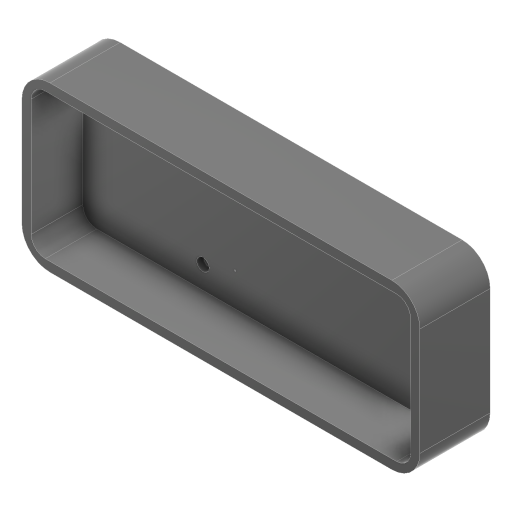
# Autodesk Inventor part: CASE_0
Saved by Autodesk Inventor 2023.2 (Build 272271000, 271)
## iProperties
Created: 2023-06-14
Part Number: CASE_0
Material: Generic
Document SubType Name: Modeling
Designer: samdi
Density: 1 g/cm^3
Appearance: Smooth - Black
Author: samdi
Autodesk Inventor part; units mm, degrees
ref_plane "YZ Plane" through (0, 0, 0) normal (1, 0, 0) x (0, 1, 0)
ref_plane "XZ Plane" through (0, 0, 0) normal (0, 1, 0) x (-1, 0, 0)
ref_plane "XY Plane" through (0, 0, 0) normal (0, 0, 1) x (1, 0, 0)
sketch "Sketch1" plane through (0, 0, 0) normal (0, 0, 1) x (1, 0, 0)
  line L0 (-16.1167, 9.6221) -> (-16.0287, 9.5557)
  line L1 (-16.2227, 9.6523) -> (-16.1167, 9.6221)
  line L2 (-16.3325, 9.6421) -> (-16.2227, 9.6523)
  line L3 (-16.4312, 9.593) -> (-16.3325, 9.6421)
  line L4 (-16.5055, 9.5115) -> (-16.4312, 9.593)
  line L5 (-16.0287, 9.5557) -> (-15.9707, 9.4619)
  line L6 (37.1652, -14.1251) -> (-36.8348, -14.1251)
  line L7 (37.1652, -14.1251) -> (-36.8348, -14.1251)
  line L8 (-13.126, 14.2536) -> (37.1652, 14.2536)
  line L9 (-13.126, 14.2536) -> (37.1652, 14.2536)
  circle A0 centre (21.1652, 10.2536) radius 1.35
  circle A1 centre (21.1652, 10.2536) radius 1.35
  line L10 (40.1652, 11.2536) -> (40.1652, -11.1251)
  line L11 (40.1652, 11.2536) -> (40.1652, -11.1251)
  line L12 (40.1463, 11.5895) -> (40.1652, 11.2536)
  line L13 (40.1463, 11.5895) -> (40.1652, 11.2536)
  line L14 (-16.4721, 8.3515) -> (-16.5301, 8.4452)
  line L15 (-16.4721, 8.3515) -> (-16.5301, 8.4452)
  line L16 (-15.971, 13.4619) -> (-15.9507, 13.3536)
  line L17 (-16.5507, 13.3536) -> (-16.5456, 13.4087)
  line L18 (-16.5507, 13.3536) -> (-16.5456, 13.4087)
  line L19 (-15.971, 13.4619) -> (-15.9507, 13.3536)
  line L20 (-16.5456, 13.4087) -> (-16.5058, 13.5115)
  line L21 (-16.5456, 13.4087) -> (-16.5058, 13.5115)
  line L22 (-16.029, 13.5557) -> (-15.971, 13.4619)
  line L23 (-16.029, 13.5557) -> (-15.971, 13.4619)
  line L24 (-16.117, 13.6221) -> (-16.029, 13.5557)
  line L25 (-16.117, 13.6221) -> (-16.029, 13.5557)
  line L26 (-16.223, 13.6523) -> (-16.117, 13.6221)
  line L27 (-16.223, 13.6523) -> (-16.117, 13.6221)
  line L28 (-16.3328, 13.6421) -> (-16.223, 13.6523)
  line L29 (-16.3328, 13.6421) -> (-16.223, 13.6523)
  line L30 (-16.5058, 13.5115) -> (-16.4315, 13.593)
  line L31 (-16.4315, 13.593) -> (-16.3328, 13.6421)
  line L32 (-16.4315, 13.593) -> (-16.3328, 13.6421)
  line L33 (-16.5058, 13.5115) -> (-16.4315, 13.593)
  line L34 (-39.1803, -12.9956) -> (-39.375, -12.7212)
  line L35 (-38.9562, -13.2464) -> (-39.1803, -12.9956)
  line L36 (-38.9562, -13.2464) -> (-39.1803, -12.9956)
  line L37 (-38.7053, -13.4706) -> (-38.9562, -13.2464)
  line L38 (-38.7053, -13.4706) -> (-38.9562, -13.2464)
  line L39 (-38.4309, -13.6653) -> (-38.7053, -13.4706)
  line L40 (-38.4309, -13.6653) -> (-38.7053, -13.4706)
  line L41 (-38.1365, -13.828) -> (-38.4309, -13.6653)
  line L42 (-38.1365, -13.828) -> (-38.4309, -13.6653)
  line L43 (-37.8257, -13.9568) -> (-38.1365, -13.828)
  line L44 (-37.8257, -13.9568) -> (-38.1365, -13.828)
  line L45 (-37.5024, -14.0499) -> (-37.8257, -13.9568)
  line L46 (-37.5024, -14.0499) -> (-37.8257, -13.9568)
  line L47 (-37.1707, -14.1062) -> (-37.5024, -14.0499)
  line L48 (-37.1707, -14.1062) -> (-37.5024, -14.0499)
  line L49 (-36.8348, -14.1251) -> (-37.1707, -14.1062)
  line L50 (-36.8348, -14.1251) -> (-37.1707, -14.1062)
  line L51 (-39.1803, -12.9956) -> (-39.375, -12.7212)
  line L52 (-27.681, 12.0452) -> (-27.7013, 12.1536)
  line L53 (-27.1013, 12.1536) -> (-27.1064, 12.0984)
  line L54 (-27.1013, 12.1536) -> (-27.1064, 12.0984)
  line L55 (-27.681, 12.0452) -> (-27.7013, 12.1536)
  line L56 (-27.1064, 12.0984) -> (-27.1462, 11.9956)
  line L57 (-27.1064, 12.0984) -> (-27.1462, 11.9956)
  line L58 (-27.623, 11.9515) -> (-27.681, 12.0452)
  line L59 (-27.623, 11.9515) -> (-27.681, 12.0452)
  line L60 (-27.535, 11.885) -> (-27.623, 11.9515)
  line L61 (-27.535, 11.885) -> (-27.623, 11.9515)
  line L62 (-27.429, 11.8548) -> (-27.535, 11.885)
  line L63 (-27.429, 11.8548) -> (-27.535, 11.885)
  line L64 (-27.1462, 11.9956) -> (-27.2205, 11.9142)
  line L65 (-27.3192, 11.865) -> (-27.429, 11.8548)
  line L66 (-27.3192, 11.865) -> (-27.429, 11.8548)
  line L67 (-27.2205, 11.9142) -> (-27.3192, 11.865)
  line L68 (-27.2205, 11.9142) -> (-27.3192, 11.865)
  line L69 (-27.1462, 11.9956) -> (-27.2205, 11.9142)
  line L70 (-27.7013, 12.1536) -> (-27.7013, 13.3536)
  line L71 (-27.1013, 13.3536) -> (-27.1013, 12.1536)
  line L72 (-27.7013, 12.1536) -> (-27.7013, 13.3536)
  line L73 (-27.1013, 13.3536) -> (-27.1013, 12.1536)
  line L74 (-27.7013, 13.3536) -> (-27.6962, 13.4087)
  line L75 (-27.7013, 13.3536) -> (-27.6962, 13.4087)
  line L76 (-27.1216, 13.4619) -> (-27.1013, 13.3536)
  line L77 (-27.1216, 13.4619) -> (-27.1013, 13.3536)
  line L78 (-27.6962, 13.4087) -> (-27.6564, 13.5115)
  line L79 (-27.6962, 13.4087) -> (-27.6564, 13.5115)
  line L80 (-27.1796, 13.5557) -> (-27.1216, 13.4619)
  line L81 (-27.1796, 13.5557) -> (-27.1216, 13.4619)
  line L82 (-27.2676, 13.6221) -> (-27.1796, 13.5557)
  line L83 (-27.2676, 13.6221) -> (-27.1796, 13.5557)
  line L84 (-27.6564, 13.5115) -> (-27.5821, 13.593)
  line L85 (-27.6564, 13.5115) -> (-27.5821, 13.593)
  line L86 (-27.5821, 13.593) -> (-27.4834, 13.6421)
  line L87 (-27.5821, 13.593) -> (-27.4834, 13.6421)
  line L88 (-27.4834, 9.6421) -> (-27.3736, 9.6523)
  line L89 (-27.4834, 9.6421) -> (-27.3736, 9.6523)
  line L90 (-27.3736, 9.6523) -> (-27.2676, 9.6221)
  line L91 (-27.6564, 9.5115) -> (-27.5821, 9.593)
  line L92 (-27.6962, 9.4087) -> (-27.6564, 9.5115)
  line L93 (-27.3736, 9.6523) -> (-27.2676, 9.6221)
  line L94 (-16.5507, 12.1536) -> (-16.5507, 13.3536)
  line L95 (-16.5304, 12.0452) -> (-16.5507, 12.1536)
  line L96 (-16.4724, 11.9515) -> (-16.5304, 12.0452)
  line L97 (-15.9507, 13.3536) -> (-15.9507, 12.1536)
  line L98 (-15.9507, 12.1536) -> (-15.9558, 12.0984)
  line L99 (-16.5507, 12.1536) -> (-16.5507, 13.3536)
  line L100 (-15.9507, 13.3536) -> (-15.9507, 12.1536)
  line L101 (-15.9507, 12.1536) -> (-15.9558, 12.0984)
  line L102 (-16.5304, 12.0452) -> (-16.5507, 12.1536)
  line L103 (-15.9558, 12.0984) -> (-15.9956, 11.9956)
  line L104 (-16.3844, 11.885) -> (-16.4724, 11.9515)
  line L105 (-16.3844, 11.885) -> (-16.4724, 11.9515)
  line L106 (-16.2784, 11.8548) -> (-16.3844, 11.885)
  line L107 (-16.2784, 11.8548) -> (-16.3844, 11.885)
  line L108 (-16.1686, 11.865) -> (-16.2784, 11.8548)
  line L109 (-16.1686, 11.865) -> (-16.2784, 11.8548)
  line L110 (-15.9956, 11.9956) -> (-16.0699, 11.9142)
  line L111 (-15.9956, 11.9956) -> (-16.0699, 11.9142)
  line L112 (-16.0699, 11.9142) -> (-16.1686, 11.865)
  line L113 (-16.0699, 11.9142) -> (-16.1686, 11.865)
  line L114 (-15.9558, 12.0984) -> (-15.9956, 11.9956)
  line L115 (-15.9504, 8.5536) -> (-15.9555, 8.4984)
  line L116 (-15.9504, 9.3536) -> (-15.9504, 8.5536)
  line L117 (-15.9707, 9.4619) -> (-15.9504, 9.3536)
  line L118 (-16.0287, 9.5557) -> (-15.9707, 9.4619)
  line L119 (-16.1167, 9.6221) -> (-16.0287, 9.5557)
  line L120 (-16.2227, 9.6523) -> (-16.1167, 9.6221)
  line L121 (-16.5453, 9.4087) -> (-16.5055, 9.5115)
  line L122 (-16.5504, 9.3536) -> (-16.5453, 9.4087)
  line L123 (-16.5504, 8.5536) -> (-16.5504, 9.3536)
  line L124 (-16.3325, 9.6421) -> (-16.2227, 9.6523)
  line L125 (-16.4312, 9.593) -> (-16.3325, 9.6421)
  line L126 (-15.9707, 9.4619) -> (-15.9504, 9.3536)
  line L127 (-15.9504, 9.3536) -> (-15.9504, 8.5536)
  line L128 (-15.9504, 8.5536) -> (-15.9555, 8.4984)
  line L129 (-16.5055, 9.5115) -> (-16.4312, 9.593)
  line L130 (-16.5453, 9.4087) -> (-16.5055, 9.5115)
  line L131 (-16.5504, 9.3536) -> (-16.5453, 9.4087)
  line L132 (-16.5504, 8.5536) -> (-16.5504, 9.3536)
  line L133 (-17.226, 8.4536) -> (-17.226, 14.2536)
  line L134 (-26.426, 14.2536) -> (-26.426, 8.4536)
  line L135 (-26.426, 14.2536) -> (-26.426, 8.4536)
  line L136 (-17.226, 8.4536) -> (-17.226, 14.2536)
  line L137 (-17.226, 14.2536) -> (-13.126, 14.2536)
  line L138 (-17.226, 14.2536) -> (-13.126, 14.2536)
  line L139 (-16.4724, 11.9515) -> (-16.5304, 12.0452)
  line L140 (-26.426, 8.4536) -> (-17.226, 8.4536)
  line L141 (-26.426, 8.4536) -> (-17.226, 8.4536)
  circle A2 centre (-14.8348, -10.7464) radius 1.35
  circle A3 centre (-14.8348, -10.7464) radius 1.35
  circle A4 centre (-35.8348, 10.2536) radius 1.35
  line L142 (-37.5024, 14.1784) -> (-37.1707, 14.2347)
  line L143 (-37.8257, 14.0852) -> (-37.5024, 14.1784)
  line L144 (-36.8348, 14.2536) -> (-29.926, 14.2536)
  line L145 (-36.8348, 14.2536) -> (-29.926, 14.2536)
  circle A5 centre (-35.8348, 10.2536) radius 1.35
  line L146 (-37.1707, 14.2347) -> (-36.8348, 14.2536)
  line L147 (-37.1707, 14.2347) -> (-36.8348, 14.2536)
  line L148 (-37.5024, 14.1784) -> (-37.1707, 14.2347)
  line L149 (-37.8257, 14.0852) -> (-37.5024, 14.1784)
  line L150 (-27.681, 8.4452) -> (-27.7013, 8.5536)
  line L151 (-27.7013, 8.5536) -> (-27.7013, 9.3536)
  line L152 (-27.1216, 9.4619) -> (-27.1013, 9.3536)
  line L153 (-27.1013, 9.3536) -> (-27.1013, 8.5536)
  line L154 (-27.1796, 9.5557) -> (-27.1216, 9.4619)
  line L155 (-27.1013, 8.5536) -> (-27.1064, 8.4984)
  line L156 (-27.1064, 8.4984) -> (-27.1462, 8.3956)
  line L157 (-27.2676, 9.6221) -> (-27.1796, 9.5557)
  line L158 (-27.7013, 9.3536) -> (-27.6962, 9.4087)
  line L159 (-27.5821, 9.593) -> (-27.4834, 9.6421)
  line L160 (-27.2676, 9.6221) -> (-27.1796, 9.5557)
  line L161 (-27.6564, 9.5115) -> (-27.5821, 9.593)
  line L162 (-27.1796, 9.5557) -> (-27.1216, 9.4619)
  line L163 (-27.6962, 9.4087) -> (-27.6564, 9.5115)
  line L164 (-27.1216, 9.4619) -> (-27.1013, 9.3536)
  line L165 (-27.7013, 9.3536) -> (-27.6962, 9.4087)
  line L166 (-27.1013, 9.3536) -> (-27.1013, 8.5536)
  line L167 (-27.7013, 8.5536) -> (-27.7013, 9.3536)
  line L168 (-27.681, 8.4452) -> (-27.7013, 8.5536)
  line L169 (-27.623, 8.3515) -> (-27.681, 8.4452)
  line L170 (-27.623, 8.3515) -> (-27.681, 8.4452)
  line L171 (-27.5821, 9.593) -> (-27.4834, 9.6421)
  line L172 (-27.1064, 8.4984) -> (-27.1462, 8.3956)
  line L173 (-27.1462, 8.3956) -> (-27.2205, 8.3142)
  line L174 (-27.1462, 8.3956) -> (-27.2205, 8.3142)
  line L175 (-27.535, 8.285) -> (-27.623, 8.3515)
  line L176 (-27.535, 8.285) -> (-27.623, 8.3515)
  line L177 (-27.2205, 8.3142) -> (-27.3192, 8.265)
  line L178 (-27.2205, 8.3142) -> (-27.3192, 8.265)
  line L179 (-27.429, 8.2548) -> (-27.535, 8.285)
  line L180 (-27.429, 8.2548) -> (-27.535, 8.285)
  line L181 (-27.3192, 8.265) -> (-27.429, 8.2548)
  line L182 (-27.3192, 8.265) -> (-27.429, 8.2548)
  line L183 (-27.1013, 8.5536) -> (-27.1064, 8.4984)
  line L184 (-27.3736, 13.6523) -> (-27.2676, 13.6221)
  line L185 (-27.4834, 13.6421) -> (-27.3736, 13.6523)
  line L186 (-27.4834, 13.6421) -> (-27.3736, 13.6523)
  line L187 (-29.926, 14.2536) -> (-26.426, 14.2536)
  line L188 (-29.926, 14.2536) -> (-26.426, 14.2536)
  line L189 (-27.3736, 13.6523) -> (-27.2676, 13.6221)
  circle A6 centre (-7.9777, -8.4364) radius 0.15
  circle A7 centre (-7.9777, -8.4364) radius 0.15
  line L190 (-15.9555, 8.4984) -> (-15.9953, 8.3956)
  line L191 (-15.9555, 8.4984) -> (-15.9953, 8.3956)
  line L192 (-15.9953, 8.3956) -> (-16.0696, 8.3142)
  line L193 (-15.9953, 8.3956) -> (-16.0696, 8.3142)
  line L194 (-16.0696, 8.3142) -> (-16.1683, 8.265)
  line L195 (-16.0696, 8.3142) -> (-16.1683, 8.265)
  line L196 (-16.1683, 8.265) -> (-16.2781, 8.2548)
  line L197 (-16.1683, 8.265) -> (-16.2781, 8.2548)
  line L198 (-16.2781, 8.2548) -> (-16.3841, 8.285)
  line L199 (-16.2781, 8.2548) -> (-16.3841, 8.285)
  line L200 (-16.3841, 8.285) -> (-16.4721, 8.3515)
  line L201 (-16.3841, 8.285) -> (-16.4721, 8.3515)
  line L202 (-16.5301, 8.4452) -> (-16.5504, 8.5536)
  line L203 (-16.5301, 8.4452) -> (-16.5504, 8.5536)
  line L204 (-39.8348, -11.1251) -> (-39.8348, 11.2536)
  line L205 (-39.8348, -11.1251) -> (-39.8348, 11.2536)
  line L206 (39.0356, 13.5991) -> (39.2865, 13.3749)
  line L207 (39.0356, 13.5991) -> (39.2865, 13.3749)
  line L208 (38.7613, 13.7937) -> (39.0356, 13.5991)
  line L209 (38.7613, 13.7937) -> (39.0356, 13.5991)
  line L210 (38.4668, 13.9565) -> (38.7613, 13.7937)
  line L211 (38.4668, 13.9565) -> (38.7613, 13.7937)
  line L212 (38.156, 14.0852) -> (38.4668, 13.9565)
  line L213 (38.156, 14.0852) -> (38.4668, 13.9565)
  line L214 (37.8327, 14.1784) -> (38.156, 14.0852)
  line L215 (37.8327, 14.1784) -> (38.156, 14.0852)
  line L216 (37.5011, 14.2347) -> (37.8327, 14.1784)
  line L217 (37.5011, 14.2347) -> (37.8327, 14.1784)
  line L218 (37.1652, 14.2536) -> (37.5011, 14.2347)
  line L219 (37.1652, 14.2536) -> (37.5011, 14.2347)
  line L220 (39.2865, 13.3749) -> (39.5107, 13.124)
  line L221 (39.2865, 13.3749) -> (39.5107, 13.124)
  line L222 (39.5107, 13.124) -> (39.7053, 12.8497)
  line L223 (39.5107, 13.124) -> (39.7053, 12.8497)
  line L224 (39.7053, 12.8497) -> (39.8681, 12.5552)
  line L225 (39.8681, 12.5552) -> (39.9968, 12.2444)
  line L226 (39.8681, 12.5552) -> (39.9968, 12.2444)
  line L227 (39.9968, 12.2444) -> (40.0899, 11.9211)
  line L228 (39.9968, 12.2444) -> (40.0899, 11.9211)
  line L229 (40.0899, 11.9211) -> (40.1463, 11.5895)
  line L230 (40.0899, 11.9211) -> (40.1463, 11.5895)
  line L231 (39.7053, 12.8497) -> (39.8681, 12.5552)
  line L232 (-39.8348, 11.2536) -> (-39.816, 11.5895)
  line L233 (-39.816, 11.5895) -> (-39.7596, 11.9211)
  line L234 (-38.1365, 13.9565) -> (-37.8257, 14.0852)
  line L235 (-38.4309, 13.7937) -> (-38.1365, 13.9565)
  line L236 (-38.7053, 13.5991) -> (-38.4309, 13.7937)
  line L237 (-38.9562, 13.3749) -> (-38.7053, 13.5991)
  line L238 (-39.1803, 13.124) -> (-38.9562, 13.3749)
  line L239 (-39.375, 12.8497) -> (-39.1803, 13.124)
  line L240 (-39.5377, 12.5552) -> (-39.375, 12.8497)
  line L241 (-39.6665, 12.2444) -> (-39.5377, 12.5552)
  line L242 (-39.7596, 11.9211) -> (-39.6665, 12.2444)
  line L243 (-38.1365, 13.9565) -> (-37.8257, 14.0852)
  line L244 (-38.4309, 13.7937) -> (-38.1365, 13.9565)
  line L245 (-38.7053, 13.5991) -> (-38.4309, 13.7937)
  line L246 (-38.9562, 13.3749) -> (-38.7053, 13.5991)
  line L247 (-39.1803, 13.124) -> (-38.9562, 13.3749)
  line L248 (-39.375, 12.8497) -> (-39.1803, 13.124)
  line L249 (-39.5377, 12.5552) -> (-39.375, 12.8497)
  line L250 (-39.6665, 12.2444) -> (-39.5377, 12.5552)
  line L251 (-39.7596, 11.9211) -> (-39.6665, 12.2444)
  line L252 (-39.8348, 11.2536) -> (-39.816, 11.5895)
  line L253 (-39.816, 11.5895) -> (-39.7596, 11.9211)
  line L254 (-39.5377, -12.4268) -> (-39.6665, -12.1159)
  line L255 (-39.375, -12.7212) -> (-39.5377, -12.4268)
  line L256 (-39.375, -12.7212) -> (-39.5377, -12.4268)
  line L257 (-39.5377, -12.4268) -> (-39.6665, -12.1159)
  line L258 (-39.6665, -12.1159) -> (-39.7596, -11.7927)
  line L259 (-39.7596, -11.7927) -> (-39.816, -11.461)
  line L260 (-39.7596, -11.7927) -> (-39.816, -11.461)
  line L261 (-39.816, -11.461) -> (-39.8348, -11.1251)
  line L262 (-39.816, -11.461) -> (-39.8348, -11.1251)
  line L263 (-39.6665, -12.1159) -> (-39.7596, -11.7927)
  line L264 (37.5011, -14.1062) -> (37.1652, -14.1251)
  line L265 (38.7613, -13.6653) -> (38.4668, -13.828)
  line L266 (38.7613, -13.6653) -> (38.4668, -13.828)
  line L267 (39.5107, -12.9956) -> (39.2865, -13.2464)
  line L268 (39.9968, -12.1159) -> (39.8681, -12.4268)
  line L269 (40.1652, -11.1251) -> (40.1463, -11.461)
  line L270 (40.1652, -11.1251) -> (40.1463, -11.461)
  line L271 (40.1463, -11.461) -> (40.0899, -11.7927)
  line L272 (40.1463, -11.461) -> (40.0899, -11.7927)
  line L273 (40.0899, -11.7927) -> (39.9968, -12.1159)
  line L274 (40.0899, -11.7927) -> (39.9968, -12.1159)
  line L275 (39.9968, -12.1159) -> (39.8681, -12.4268)
  line L276 (39.8681, -12.4268) -> (39.7053, -12.7212)
  line L277 (39.8681, -12.4268) -> (39.7053, -12.7212)
  line L278 (39.7053, -12.7212) -> (39.5107, -12.9956)
  line L279 (39.7053, -12.7212) -> (39.5107, -12.9956)
  line L280 (39.5107, -12.9956) -> (39.2865, -13.2464)
  line L281 (39.2865, -13.2464) -> (39.0356, -13.4706)
  line L282 (39.2865, -13.2464) -> (39.0356, -13.4706)
  line L283 (39.0356, -13.4706) -> (38.7613, -13.6653)
  line L284 (39.0356, -13.4706) -> (38.7613, -13.6653)
  line L285 (38.4668, -13.828) -> (38.156, -13.9568)
  line L286 (38.4668, -13.828) -> (38.156, -13.9568)
  line L287 (38.156, -13.9568) -> (37.8327, -14.0499)
  line L288 (37.8327, -14.0499) -> (37.5011, -14.1062)
  line L289 (37.8327, -14.0499) -> (37.5011, -14.1062)
  line L290 (37.5011, -14.1062) -> (37.1652, -14.1251)
  line L291 (38.156, -13.9568) -> (37.8327, -14.0499)
  line L292 (-36.5, 17.5) -> (36.5, 17.5)
  line L293 (42.5, 11.5) -> (42.5, -11.5)
  line L294 (36.5, -17.5) -> (-36.5, -17.5)
  line L295 (-42.5, -11.5) -> (-42.5, 11.5)
  line L296 (-42.5, 17.5) -> (42.5, -17.5) construction
  line L297 (42.5, 17.5) -> (-42.5, -17.5) construction
  arc A8 (-36.5, 17.5) -> (-42.5, 11.5) centre (-36.5, 11.5) ccw
  arc A9 (-42.5, -11.5) -> (-36.5, -17.5) centre (-36.5, -11.5) ccw
  arc A10 (36.5, -17.5) -> (42.5, -11.5) centre (36.5, -11.5) ccw
  arc A11 (42.5, 11.5) -> (36.5, 17.5) centre (36.5, 11.5) ccw
  line L298 (37.5, 15.5) -> (-37.5, 15.5)
  line L299 (-40.5, 12.5) -> (-40.5, -12.5)
  line L300 (-37.5, -15.5) -> (37.5, -15.5)
  line L301 (40.5, -12.5) -> (40.5, 12.5)
  line L302 (40.5, 15.5) -> (-40.5, -15.5) construction
  line L303 (-40.5, 15.5) -> (40.5, -15.5) construction
  arc A12 (-40.5, -12.5) -> (-37.5, -15.5) centre (-37.5, -12.5) ccw
  arc A13 (-37.5, 15.5) -> (-40.5, 12.5) centre (-37.5, 12.5) ccw
  arc A14 (40.5, 12.5) -> (37.5, 15.5) centre (37.5, 12.5) ccw
  arc A15 (37.5, -15.5) -> (40.5, -12.5) centre (37.5, -12.5) ccw
  point P0 (0, 0)
  dimension "d2" = 85
  dimension "d3" = 35
  dimension "d4" = 6
  dimension "d5" = 81
  dimension "d6" = 31
  dimension "d7" = 3
  dimension "d8" = 3
  constraints: 608 end point, 16 centre point, 16 point on circle, 16 point on line, 16 tangent, 5 equal radius, 4 midpoint, 4 parallel, 2 horizontal, 2 perpendicular
  measures "d2" distance of L296.end L297.end
  measures "d3" distance of L297.start L296.end
  measures "d4" radius of A8
  measures "d5" distance of L303.end L302.end
  measures "d6" distance of L302.end L303.start
  measures "d7" radius of A12
  measures "d8" radius of A13
extrude "Extrusion1" add sketch "Sketch1" along normal blind 2.5 contours L0 L5 L117 L116 L115 L190 L192 L194 L196 L198 L200 L14 L202 L123 L122 L121 L4 L3 L2 L1 | L6 L49 L47 L45 L43 L41 L39 L37 L35 L34 L255 L254 L258 L259 L261 L204 L232 L233 L242 L241 L240 L239 L238 L237 L236 L235 L234 L143 L142 L146 L144 L187 L134 L140 L133 L137 L8 L218 L216 L214 L212 L210 L208 L206 L220 L222 L224 L225 L227 L229 L12 L10 L269 L271 L273 L268 L276 L278 L267 L281 L283 L265 L285 L287 L288 L264 | A0 | L16 L97 L98 L103 L110 L112 L108 L106 L104 L96 L95 L94 L17 L20 L30 L31 L28 L26 L24 L22 | L52 L70 L74 L78 L84 L86 L185 L184 L82 L80 L76 L71 L53 L56 L64 L67 L65 L62 L60 L58 | L88 L90 L157 L154 L152 L153 L155 L156 L173 L177 L181 L179 L175 L169 L150 L151 L158 L92 L91 L159 | A2 | A4 | A6 | L292 A11 L293 A10 L294 A9 L295 A8 | A14 L301 A15 L300 A12 L299 A13 L298
extrude "Extrusion2" add sketch "Sketch1" along normal blind 15 contours L292 A11 L293 A10 L294 A9 L295 A8
extrude "Extrusion3" add sketch "Sketch1" along normal blind 4 contours L0 L5 L117 L116 L115 L190 L192 L194 L196 L198 L200 L14 L202 L123 L122 L121 L4 L3 L2 L1 | L6 L49 L47 L45 L43 L41 L39 L37 L35 L34 L255 L254 L258 L259 L261 L204 L232 L233 L242 L241 L240 L239 L238 L237 L236 L235 L234 L143 L142 L146 L144 L187 L134 L140 L133 L137 L8 L218 L216 L214 L212 L210 L208 L206 L220 L222 L224 L225 L227 L229 L12 L10 L269 L271 L273 L268 L276 L278 L267 L281 L283 L265 L285 L287 L288 L264 | L16 L97 L98 L103 L110 L112 L108 L106 L104 L96 L95 L94 L17 L20 L30 L31 L28 L26 L24 L22 | L52 L70 L74 L78 L84 L86 L185 L184 L82 L80 L76 L71 L53 L56 L64 L67 L65 L62 L60 L58 | L88 L90 L157 L154 L152 L153 L155 L156 L173 L177 L181 L179 L175 L169 L150 L151 L158 L92 L91 L159 | A14 L301 A15 L300 A12 L299 A13 L298
sketch "Sketch3" plane through (0, 0, 15) normal (0, 0, 1) x (1, 0, 0)
  line L0 (-36.5, -17.5) -> (36.5, -17.5) projected
  arc A0 (36.5, -17.5) -> (42.5, -11.5) centre (36.5, -11.5) ccw projected
  line L1 (42.5, -11.5) -> (42.5, 11.5) projected
  arc A1 (42.5, 11.5) -> (36.5, 17.5) centre (36.5, 11.5) ccw projected
  line L2 (36.5, 17.5) -> (-36.5, 17.5) projected
  arc A2 (-36.5, 17.5) -> (-42.5, 11.5) centre (-36.5, 11.5) ccw projected
  line L3 (-42.5, 11.5) -> (-42.5, -11.5) projected
  arc A3 (-42.5, -11.5) -> (-36.5, -17.5) centre (-36.5, -11.5) ccw projected
  arc A4 (40.5, 12.5) -> (37.5, 15.5) centre (37.5, 12.5) ccw projected
  line L4 (40.5, 12.5) -> (40.5, -12.5) projected
  arc A5 (37.5, -15.5) -> (40.5, -12.5) centre (37.5, -12.5) ccw projected
  line L5 (37.5, -15.5) -> (-37.5, -15.5) projected
  arc A6 (-40.5, -12.5) -> (-37.5, -15.5) centre (-37.5, -12.5) ccw projected
  line L6 (-40.5, -12.5) -> (-40.5, 12.5) projected
  arc A7 (-37.5, 15.5) -> (-40.5, 12.5) centre (-37.5, 12.5) ccw projected
  line L7 (-37.5, 15.5) -> (37.5, 15.5) projected
  point P0 (0, 0)
body "Solid1"
